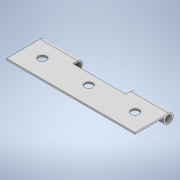
# Autodesk Inventor part: Ala 1 Bisagra tipo Libro Chica
Saved by Autodesk Inventor 2020 (Build 240168000, 168)
## iProperties
Created: 2020-06-18
Part Number: Ala 1 Bisagra tipo Libro Chica
Material: Genérico
Document SubType Name: Modeling
Designer: Pipi
Density: 1 g/cm^3
Appearance: Valor por defecto
Author: Pipi
Autodesk Inventor part; units mm, degrees
ref_plane "YZ Plane" through (0, 0, 0) normal (1, 0, 0) x (0, 1, 0)
ref_plane "XZ Plane" through (0, 0, 0) normal (0, 1, 0) x (-1, 0, 0)
ref_plane "XY Plane" through (0, 0, 0) normal (0, 0, 1) x (1, 0, 0)
sketch "Boceto1" plane through (0, 0, 0) normal (0, 1, 0) x (-1, 0, 0)
  line L0 (6.207, 40.007) -> (6.207, 26.007)
  line L1 (6.207, 26.007) -> (-56.793, 26.007)
  line L2 (-56.793, 26.007) -> (-56.793, 40.007)
  line L3 (-56.793, 40.007) -> (6.207, 40.007)
  circle A0 centre (-2.543, 31.257) radius 2
  circle A1 centre (-48.043, 31.257) radius 2
  circle A2 centre (-25.293, 31.257) radius 2
  point P0 (0, 0)
  dimension "d0" = 14
  dimension "d1" = 63
  dimension "d33" = 4
  dimension "d34" = 4
  dimension "d35" = 4
  dimension "d36" = 8.75
  dimension "d37" = 8.75
  dimension "d38" = 8.75
  dimension "d39" = 8.75
  dimension "d40" = 8.75
  dimension "d41" = 31.5
  constraints: 8 end point, 3 centre point, 3 perpendicular, 1 vertical
  measures "d0" distance of L0.start L0.end
  measures "d1" distance of L0.end L1.end
  measures "d33" diameter of A0
  measures "d34" diameter of A1
  measures "d35" diameter of A2
  measures "d36" distance from line of L3 A0.centre
  measures "d37" distance from line of L3 A2.centre
  measures "d38" distance from line of L3 A1.centre
  measures "d39" distance from line of L2 A1.centre
  measures "d40" distance from line of L0 A0.centre
  measures "d41" distance from line of L0 A2.centre
extrude "Extrusión1" add sketch "Boceto1" along normal blind 0.8
sketch "Boceto7" plane through (56.793, 0, 40.007) normal (1, 0, 0) x (0, 0, -1)
  circle A0 centre (16.375, -1.575) radius 2.375
  circle A1 centre (16.375, -1.575) radius 1.625
  line L0 (14, 0) -> (14, 0.8) projected
  line L1 (0, 0.8) -> (14, 0.8) projected
  line L2 (0, 0) -> (14, 0) projected
  line L3 (14, 0) -> (14, -1.575)
  line L4 (14, 0.8) -> (16.375, 0.8)
  line L5 (14, 0.8) -> (14, 0)
  point P0 (40.007, 0)
  dimension "d25" = 4.75
  dimension "d26" = 3.25
  constraints: 6 end point, 3 tangent, 2 centre point, 2 perpendicular, 2 point on circle, 1 coincident
  measures "d25" diameter of A0
  measures "d26" diameter of A1
extrude "Extrusión4" add sketch "Boceto7" against normal blind 63
sketch "Boceto9" plane through (0, 0.8, 0) normal (0, 1, 0) x (1, 0, 0)
  line L0 (-6.207, -25.257) -> (56.793, -25.257) projected
  line L1 (-6.207, -40.007) -> (-6.207, -23.632) projected
  line L2 (12.293, -25.007) -> (12.293, -15.007)
  line L3 (12.293, -15.007) -> (38.2918, -15.007)
  line L4 (38.2918, -15.007) -> (38.2918, -25.257)
  line L5 (38.2918, -25.257) -> (38.2918, -26.007)
  line L6 (56.793, -26.007) -> (-6.207, -26.007) projected
  line L7 (12.293, -25.007) -> (12.293, -26.007)
  line L8 (12.293, -26.007) -> (38.2918, -26.007)
  line L9 (56.793, -25.257) -> (38.2918, -25.257)
  line L10 (12.293, -25.007) -> (-6.207, -25.007)
  point P0 (0, 0)
  point P1 (38.2918, -25.257)
  point P2 (12.293, -25.257)
  point P3 (38.2918, -25.257)
  dimension "d43" = 26
  constraints: 16 end point, 4 perpendicular, 3 point on line, 2 horizontal, 2 vertical
  measures "d43" distance of L4.end L2.start
extrude "Extrusión6" cut sketch "Boceto9" against normal blind 63 contours L7 L2 L3 L4 L0 | L0 L5 L6 L7
